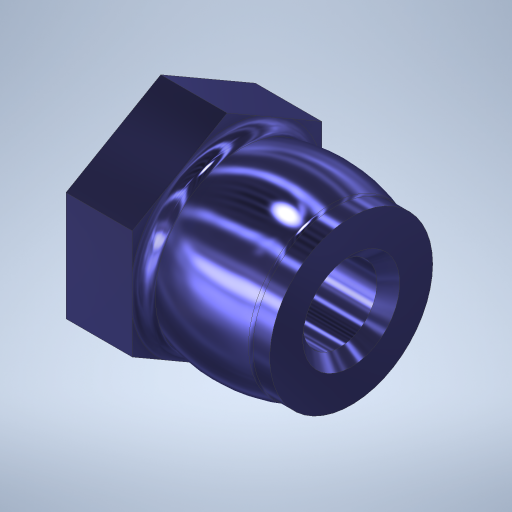
# Autodesk Inventor part: Shock Bushing
Saved by Autodesk Inventor 2023.1 (Build 271208000, 208)
## iProperties
Created: 2019-11-28
Part Number: Shock Bushing
Material: Generic
Document SubType Name: Modeling
Designer: Jopa
Density: 1 g/cm^3
Appearance: Default
Author: Jopa
Autodesk Inventor part; units mm, degrees
ref_plane "YZ Plane" through (0, 0, 0) normal (1, 0, 0) x (0, 1, 0)
ref_plane "XZ Plane" through (0, 0, 0) normal (0, 1, 0) x (-1, 0, 0)
ref_plane "XY Plane" through (0, 0, 0) normal (0, 0, 1) x (1, 0, 0)
sketch "Sketch1" plane through (0, 0, 0) normal (0, 0, 1) x (1, 0, 0)
  line L0 (-6.9037, 0) -> (1.1506, 0) projected
  line L1 (0, -3.0734) -> (0, 4.2164) construction
  line L2 (-3.5306, 3.175) -> (-5.7531, 3.175)
  line L3 (-5.7531, 3.175) -> (-5.7531, 1.2446)
  line L4 (-5.7531, 1.2446) -> (0, 1.2446)
  line L5 (0, 1.2446) -> (0, 2.7314)
  line L6 (-3.5306, 3.175) -> (-3.5306, 2.7314)
  arc A0 (0, 2.7314) -> (-3.5306, 2.7314) centre (-1.7653, -2.032) ccw
  point P0 (0, 0)
  dimension "d0" = 6.35
  dimension "d1" = 5.08
  dimension "d2" = 3.9878
  dimension "d3" = 2.2225
  dimension "d5" = 2.4892
  dimension "d6" = 5.4628
  constraints: 10 end point, 3 perpendicular, 2 point on circle, 1 centre point, 1 collinear, 1 horizontal, 1 horizontal alignment, 1 vertical
  measures "d0" diameter of L2 L0
  measures "d1" radius of A0
  measures "d2" distance from line of L3 A0.centre
  measures "d3" distance of L2.start L2.end
  measures "d5" diameter of L4 L0
  measures "d6" diameter of L5.end L0
revolve "Revolution1" add sketch "Sketch1" angle 360 about axis through (-10, 0, 0) along (1, 0, 0)
sketch "Sketch2" plane through (-5.7531, 0, 0) normal (-1, 0, 0) x (0, 0, 1)
  circle A0 centre (0, 0) radius 3.175 projected
  line L0 (3.175, -1.8331) -> (0, -3.6662)
  line L1 (0, -3.6662) -> (-3.175, -1.8331)
  line L2 (-3.175, -1.8331) -> (-3.175, 1.8331)
  line L3 (-3.175, 1.8331) -> (0, 3.6662)
  line L4 (0, 3.6662) -> (3.175, 1.8331)
  line L5 (3.175, 1.8331) -> (3.175, -1.8331)
  point P0 (3.175, 0)
  constraints: 12 end point, 1 coincident, 1 horizontal alignment, 1 midpoint, 1 vertical, 14 other
extrude "Extrusion1" add sketch "Sketch2" against normal up to surface (2.2225 mm away) contours L5 L0 A0 | A0 L4 L5 | A0 L3 L4 | L0 L1 A0 | A0 L2 L3 | L1 L2 A0
sketch "Sketch3" plane through (0, 0, 0) normal (1, 0, 0) x (0, 0, -1)
  circle A0 centre (0, 0) radius 2.7314 projected
  circle A1 centre (0, 0) radius 1.2446 projected
extrude "Extrusion2" add sketch "Sketch3" along normal blind 0.635
fillet "Fillet1" radius 0.381 3 edges at (-3.5306, -2.7314, 0) (0, 1.9314, -1.9314) (0, -1.9314, 1.9314)
chamfer "Chamfer1" distance 0.381 angle 45 1 edges at (0.635, 0, 1.2446)
body "Solid1"
